Autodesk Inventor part; units mm, degrees
(part 2 of 2)
sketch "草圖6" plane through (-20.1844, 0, 27.5664) normal (0, 0, 1) x (1, 0, 0)
  line L0 (95.2719, 28.2499) -> (97.7719, 28.2499)
  line L1 (97.7719, 28.2499) -> (97.7719, 23.2499)
  line L2 (97.7719, 23.2499) -> (95.2719, 23.2499)
  line L3 (95.2719, 23.2499) -> (95.2719, 28.2499)
  line L4 (95.2719, 21.2499) -> (97.7719, 21.2499)
  line L5 (95.2719, 16.2499) -> (95.2719, 21.2499)
  line L6 (97.7719, 16.2499) -> (95.2719, 16.2499)
  line L7 (97.7719, 21.2499) -> (97.7719, 16.2499)
  line L8 (95.2719, 14.2499) -> (97.7719, 14.2499)
  line L9 (95.2719, 9.2499) -> (95.2719, 14.2499)
  line L10 (97.7719, 9.2499) -> (95.2719, 9.2499)
  line L11 (97.7719, 14.2499) -> (97.7719, 9.2499)
  line L12 (95.2719, 7.2499) -> (97.7719, 7.2499)
  line L13 (95.2719, 2.2499) -> (95.2719, 7.2499)
  line L14 (97.7719, 2.2499) -> (95.2719, 2.2499)
  line L15 (97.7719, 7.2499) -> (97.7719, 2.2499)
  line L16 (92.2719, 28.2499) -> (89.7719, 28.2499)
  line L17 (89.7719, 28.2499) -> (89.7719, 23.3875)
  line L18 (89.7719, 23.3875) -> (92.2719, 23.3875)
  line L19 (92.2719, 23.3875) -> (92.2719, 28.2499)
  line L20 (88.2719, 28.2499) -> (85.7719, 28.2499)
  line L21 (85.7719, 28.2499) -> (85.7719, 23.3875)
  line L22 (85.7719, 23.3875) -> (88.2719, 23.3875)
  line L23 (88.2719, 23.3875) -> (88.2719, 28.2499)
  line L24 (92.2719, 21.2499) -> (89.7719, 21.2499)
  line L25 (89.7719, 21.2499) -> (89.7719, 16.3875)
  line L26 (89.7719, 16.3875) -> (92.2719, 16.3875)
  line L27 (92.2719, 16.3875) -> (92.2719, 21.2499)
  line L28 (88.2719, 21.2499) -> (85.7719, 21.2499)
  line L29 (85.7719, 21.2499) -> (85.7719, 16.3875)
  line L30 (85.7719, 16.3875) -> (88.2719, 16.3875)
  line L31 (88.2719, 16.3875) -> (88.2719, 21.2499)
  line L32 (92.2719, 14.2499) -> (89.7719, 14.2499)
  line L33 (89.7719, 14.2499) -> (89.7719, 9.3875)
  line L34 (89.7719, 9.3875) -> (92.2719, 9.3875)
  line L35 (92.2719, 9.3875) -> (92.2719, 14.2499)
  line L36 (88.2719, 14.2499) -> (85.7719, 14.2499)
  line L37 (85.7719, 14.2499) -> (85.7719, 9.3875)
  line L38 (85.7719, 9.3875) -> (88.2719, 9.3875)
  line L39 (88.2719, 9.3875) -> (88.2719, 14.2499)
  line L40 (92.2719, 7.2499) -> (89.7719, 7.2499)
  line L41 (89.7719, 7.2499) -> (89.7719, 2.3875)
  line L42 (89.7719, 2.3875) -> (92.2719, 2.3875)
  line L43 (92.2719, 2.3875) -> (92.2719, 7.2499)
  line L44 (88.2719, 7.2499) -> (85.7719, 7.2499)
  line L45 (85.7719, 7.2499) -> (85.7719, 2.3875)
  line L46 (85.7719, 2.3875) -> (88.2719, 2.3875)
  line L47 (88.2719, 2.3875) -> (88.2719, 7.2499)
  line L48 (78.2719, 21.2499) -> (75.7719, 21.2499)
  line L49 (75.7719, 16.3875) -> (78.2719, 16.3875)
  line L50 (75.7719, 21.2499) -> (75.7719, 16.3875)
  line L51 (78.2719, 16.3875) -> (78.2719, 21.2499)
  line L52 (79.7719, 21.2499) -> (79.7719, 16.3875)
  line L53 (79.7719, 16.3875) -> (82.2719, 16.3875)
  line L54 (82.2719, 16.3875) -> (82.2719, 21.2499)
  line L55 (82.2719, 21.2499) -> (79.7719, 21.2499)
  line L56 (78.2719, 14.2499) -> (75.7719, 14.2499)
  line L57 (79.7719, 9.3875) -> (82.2719, 9.3875)
  line L58 (75.7719, 9.3875) -> (78.2719, 9.3875)
  line L59 (75.7719, 14.2499) -> (75.7719, 9.3875)
  line L60 (79.7719, 14.2499) -> (79.7719, 9.3875)
  line L61 (82.2719, 9.3875) -> (82.2719, 14.2499)
  line L62 (78.2719, 9.3875) -> (78.2719, 14.2499)
  line L63 (82.2719, 14.2499) -> (79.7719, 14.2499)
  line L64 (82.2719, 7.2499) -> (79.7719, 7.2499)
  line L65 (78.2719, 7.2499) -> (75.7719, 7.2499)
  line L66 (79.7719, 7.2499) -> (79.7719, 2.3875)
  line L67 (82.2719, 2.3875) -> (82.2719, 7.2499)
  line L68 (78.2719, 2.3875) -> (78.2719, 7.2499)
  line L69 (75.7719, 7.2499) -> (75.7719, 2.3875)
  line L70 (75.7719, 2.3875) -> (78.2719, 2.3875)
  line L71 (79.7719, 2.3875) -> (82.2719, 2.3875)
  line L72 (79.7719, 23.3875) -> (82.2719, 23.3875)
  line L73 (82.2719, 28.2499) -> (79.7719, 28.2499)
  line L74 (82.2719, 23.3875) -> (82.2719, 28.2499)
  line L75 (79.7719, 28.2499) -> (79.7719, 23.3875)
  line L76 (75.7719, 23.3875) -> (78.2719, 23.3875)
  line L77 (78.2719, 23.3875) -> (78.2719, 28.2499)
  line L78 (75.7719, 28.2499) -> (75.7719, 23.3875)
  line L79 (78.2719, 28.2499) -> (75.7719, 28.2499)
  line L80 (68.2719, 21.2499) -> (65.7719, 21.2499)
  line L81 (65.7719, 16.3875) -> (68.2719, 16.3875)
  line L82 (65.7719, 21.2499) -> (65.7719, 16.3875)
  line L83 (68.2719, 16.3875) -> (68.2719, 21.2499)
  line L84 (69.7719, 21.2499) -> (69.7719, 16.3875)
  line L85 (69.7719, 16.3875) -> (72.2719, 16.3875)
  line L86 (72.2719, 16.3875) -> (72.2719, 21.2499)
  line L87 (72.2719, 21.2499) -> (69.7719, 21.2499)
  line L88 (68.2719, 14.2499) -> (65.7719, 14.2499)
  line L89 (69.7719, 9.3875) -> (72.2719, 9.3875)
  line L90 (65.7719, 9.3875) -> (68.2719, 9.3875)
  line L91 (65.7719, 14.2499) -> (65.7719, 9.3875)
  line L92 (69.7719, 14.2499) -> (69.7719, 9.3875)
  line L93 (72.2719, 9.3875) -> (72.2719, 14.2499)
  line L94 (68.2719, 9.3875) -> (68.2719, 14.2499)
  line L95 (72.2719, 14.2499) -> (69.7719, 14.2499)
  line L96 (72.2719, 7.2499) -> (69.7719, 7.2499)
  line L97 (68.2719, 7.2499) -> (65.7719, 7.2499)
  line L98 (69.7719, 7.2499) -> (69.7719, 2.3875)
  line L99 (72.2719, 2.3875) -> (72.2719, 7.2499)
  line L100 (68.2719, 2.3875) -> (68.2719, 7.2499)
  line L101 (65.7719, 7.2499) -> (65.7719, 2.3875)
  line L102 (65.7719, 2.3875) -> (68.2719, 2.3875)
  line L103 (69.7719, 2.3875) -> (72.2719, 2.3875)
  line L104 (69.7719, 23.3875) -> (72.2719, 23.3875)
  line L105 (72.2719, 28.2499) -> (69.7719, 28.2499)
  line L106 (72.2719, 23.3875) -> (72.2719, 28.2499)
  line L107 (69.7719, 28.2499) -> (69.7719, 23.3875)
  line L108 (65.7719, 23.3875) -> (68.2719, 23.3875)
  line L109 (68.2719, 23.3875) -> (68.2719, 28.2499)
  line L110 (65.7719, 28.2499) -> (65.7719, 23.3875)
  line L111 (68.2719, 28.2499) -> (65.7719, 28.2499)
  line L112 (60.2719, 28.2499) -> (62.7719, 28.2499)
  line L113 (62.7719, 28.2499) -> (62.7719, 23.2499)
  line L114 (62.7719, 23.2499) -> (60.2719, 23.2499)
  line L115 (60.2719, 23.2499) -> (60.2719, 28.2499)
  line L116 (100, 30) -> (0, 30) projected
  line L117 (50, 30) -> (50, 0)
  line L118 (100, 0) -> (0, 0) projected
  line L119 (52.9784, 0) -> (46.9661, 0)
  line L120 (46.9661, 0) -> (46.9661, 21.3875)
  line L121 (46.9661, 21.3875) -> (52.9784, 21.3875)
  line L122 (52.9784, 21.3875) -> (52.9784, 0)
  line L123 (60.2719, 21.2499) -> (62.7719, 21.2499)
  line L124 (60.2719, 16.2499) -> (60.2719, 21.2499)
  line L125 (62.7719, 16.2499) -> (60.2719, 16.2499)
  line L126 (62.7719, 21.2499) -> (62.7719, 16.2499)
  line L127 (60.2719, 14.2499) -> (62.7719, 14.2499)
  line L128 (60.2719, 9.2499) -> (60.2719, 14.2499)
  line L129 (62.7719, 9.2499) -> (60.2719, 9.2499)
  line L130 (62.7719, 14.2499) -> (62.7719, 9.2499)
  line L131 (60.2719, 7.2499) -> (62.7719, 7.2499)
  line L132 (60.2719, 2.2499) -> (60.2719, 7.2499)
  line L133 (62.7719, 2.2499) -> (60.2719, 2.2499)
  line L134 (62.7719, 7.2499) -> (62.7719, 2.2499)
  line L135 (4.7281, 28.2499) -> (2.2281, 28.2499)
  line L136 (2.2281, 28.2499) -> (2.2281, 23.2499)
  line L137 (2.2281, 23.2499) -> (4.7281, 23.2499)
  line L138 (4.7281, 23.2499) -> (4.7281, 28.2499)
  line L139 (4.7281, 21.2499) -> (2.2281, 21.2499)
  line L140 (4.7281, 16.2499) -> (4.7281, 21.2499)
  line L141 (2.2281, 16.2499) -> (4.7281, 16.2499)
  line L142 (2.2281, 21.2499) -> (2.2281, 16.2499)
  line L143 (4.7281, 14.2499) -> (2.2281, 14.2499)
  line L144 (4.7281, 9.2499) -> (4.7281, 14.2499)
  line L145 (2.2281, 9.2499) -> (4.7281, 9.2499)
  line L146 (2.2281, 14.2499) -> (2.2281, 9.2499)
  line L147 (4.7281, 7.2499) -> (2.2281, 7.2499)
  line L148 (4.7281, 2.2499) -> (4.7281, 7.2499)
  line L149 (2.2281, 2.2499) -> (4.7281, 2.2499)
  line L150 (2.2281, 7.2499) -> (2.2281, 2.2499)
  line L151 (7.7281, 28.2499) -> (10.2281, 28.2499)
  line L152 (10.2281, 28.2499) -> (10.2281, 23.3875)
  line L153 (10.2281, 23.3875) -> (7.7281, 23.3875)
  line L154 (7.7281, 23.3875) -> (7.7281, 28.2499)
  line L155 (11.7281, 28.2499) -> (14.2281, 28.2499)
  line L156 (14.2281, 28.2499) -> (14.2281, 23.3875)
  line L157 (14.2281, 23.3875) -> (11.7281, 23.3875)
  line L158 (11.7281, 23.3875) -> (11.7281, 28.2499)
  line L159 (7.7281, 21.2499) -> (10.2281, 21.2499)
  line L160 (10.2281, 21.2499) -> (10.2281, 16.3875)
  line L161 (10.2281, 16.3875) -> (7.7281, 16.3875)
  line L162 (7.7281, 16.3875) -> (7.7281, 21.2499)
  line L163 (11.7281, 21.2499) -> (14.2281, 21.2499)
  line L164 (14.2281, 21.2499) -> (14.2281, 16.3875)
  line L165 (14.2281, 16.3875) -> (11.7281, 16.3875)
  line L166 (11.7281, 16.3875) -> (11.7281, 21.2499)
  line L167 (7.7281, 14.2499) -> (10.2281, 14.2499)
  line L168 (10.2281, 14.2499) -> (10.2281, 9.3875)
  line L169 (10.2281, 9.3875) -> (7.7281, 9.3875)
  line L170 (7.7281, 9.3875) -> (7.7281, 14.2499)
  line L171 (11.7281, 14.2499) -> (14.2281, 14.2499)
  line L172 (14.2281, 14.2499) -> (14.2281, 9.3875)
  line L173 (14.2281, 9.3875) -> (11.7281, 9.3875)
  line L174 (11.7281, 9.3875) -> (11.7281, 14.2499)
  line L175 (7.7281, 7.2499) -> (10.2281, 7.2499)
  line L176 (10.2281, 7.2499) -> (10.2281, 2.3875)
  line L177 (10.2281, 2.3875) -> (7.7281, 2.3875)
  line L178 (7.7281, 2.3875) -> (7.7281, 7.2499)
  line L179 (11.7281, 7.2499) -> (14.2281, 7.2499)
  line L180 (14.2281, 7.2499) -> (14.2281, 2.3875)
  line L181 (14.2281, 2.3875) -> (11.7281, 2.3875)
  line L182 (11.7281, 2.3875) -> (11.7281, 7.2499)
  line L183 (21.7281, 21.2499) -> (24.2281, 21.2499)
  line L184 (24.2281, 16.3875) -> (21.7281, 16.3875)
  line L185 (24.2281, 21.2499) -> (24.2281, 16.3875)
  line L186 (21.7281, 16.3875) -> (21.7281, 21.2499)
  line L187 (20.2281, 21.2499) -> (20.2281, 16.3875)
  line L188 (20.2281, 16.3875) -> (17.7281, 16.3875)
  line L189 (17.7281, 16.3875) -> (17.7281, 21.2499)
  line L190 (17.7281, 21.2499) -> (20.2281, 21.2499)
  line L191 (21.7281, 14.2499) -> (24.2281, 14.2499)
  line L192 (20.2281, 9.3875) -> (17.7281, 9.3875)
  line L193 (24.2281, 9.3875) -> (21.7281, 9.3875)
  line L194 (24.2281, 14.2499) -> (24.2281, 9.3875)
  line L195 (20.2281, 14.2499) -> (20.2281, 9.3875)
  line L196 (17.7281, 9.3875) -> (17.7281, 14.2499)
  line L197 (21.7281, 9.3875) -> (21.7281, 14.2499)
  line L198 (17.7281, 14.2499) -> (20.2281, 14.2499)
  line L199 (17.7281, 7.2499) -> (20.2281, 7.2499)
  line L200 (21.7281, 7.2499) -> (24.2281, 7.2499)
  line L201 (20.2281, 7.2499) -> (20.2281, 2.3875)
  line L202 (17.7281, 2.3875) -> (17.7281, 7.2499)
  line L203 (21.7281, 2.3875) -> (21.7281, 7.2499)
  line L204 (24.2281, 7.2499) -> (24.2281, 2.3875)
  line L205 (24.2281, 2.3875) -> (21.7281, 2.3875)
  line L206 (20.2281, 2.3875) -> (17.7281, 2.3875)
  line L207 (20.2281, 23.3875) -> (17.7281, 23.3875)
  line L208 (17.7281, 28.2499) -> (20.2281, 28.2499)
  line L209 (17.7281, 23.3875) -> (17.7281, 28.2499)
  line L210 (20.2281, 28.2499) -> (20.2281, 23.3875)
  line L211 (24.2281, 23.3875) -> (21.7281, 23.3875)
  line L212 (21.7281, 23.3875) -> (21.7281, 28.2499)
  line L213 (24.2281, 28.2499) -> (24.2281, 23.3875)
  line L214 (21.7281, 28.2499) -> (24.2281, 28.2499)
  line L215 (31.7281, 21.2499) -> (34.2281, 21.2499)
  line L216 (34.2281, 16.3875) -> (31.7281, 16.3875)
  line L217 (34.2281, 21.2499) -> (34.2281, 16.3875)
  line L218 (31.7281, 16.3875) -> (31.7281, 21.2499)
  line L219 (30.2281, 21.2499) -> (30.2281, 16.3875)
  line L220 (30.2281, 16.3875) -> (27.7281, 16.3875)
  line L221 (27.7281, 16.3875) -> (27.7281, 21.2499)
  line L222 (27.7281, 21.2499) -> (30.2281, 21.2499)
  line L223 (31.7281, 14.2499) -> (34.2281, 14.2499)
  line L224 (30.2281, 9.3875) -> (27.7281, 9.3875)
  line L225 (34.2281, 9.3875) -> (31.7281, 9.3875)
  line L226 (34.2281, 14.2499) -> (34.2281, 9.3875)
  line L227 (30.2281, 14.2499) -> (30.2281, 9.3875)
  line L228 (27.7281, 9.3875) -> (27.7281, 14.2499)
  line L229 (31.7281, 9.3875) -> (31.7281, 14.2499)
  line L230 (27.7281, 14.2499) -> (30.2281, 14.2499)
  line L231 (27.7281, 7.2499) -> (30.2281, 7.2499)
  line L232 (31.7281, 7.2499) -> (34.2281, 7.2499)
  line L233 (30.2281, 7.2499) -> (30.2281, 2.3875)
  line L234 (27.7281, 2.3875) -> (27.7281, 7.2499)
  line L235 (31.7281, 2.3875) -> (31.7281, 7.2499)
  line L236 (34.2281, 7.2499) -> (34.2281, 2.3875)
  line L237 (34.2281, 2.3875) -> (31.7281, 2.3875)
  line L238 (30.2281, 2.3875) -> (27.7281, 2.3875)
  line L239 (30.2281, 23.3875) -> (27.7281, 23.3875)
  line L240 (27.7281, 28.2499) -> (30.2281, 28.2499)
  line L241 (27.7281, 23.3875) -> (27.7281, 28.2499)
  line L242 (30.2281, 28.2499) -> (30.2281, 23.3875)
  line L243 (34.2281, 23.3875) -> (31.7281, 23.3875)
  line L244 (31.7281, 23.3875) -> (31.7281, 28.2499)
  line L245 (34.2281, 28.2499) -> (34.2281, 23.3875)
  line L246 (31.7281, 28.2499) -> (34.2281, 28.2499)
  line L247 (39.7281, 28.2499) -> (37.2281, 28.2499)
  line L248 (37.2281, 28.2499) -> (37.2281, 23.2499)
  line L249 (37.2281, 23.2499) -> (39.7281, 23.2499)
  line L250 (39.7281, 23.2499) -> (39.7281, 28.2499)
  line L251 (39.7281, 21.2499) -> (37.2281, 21.2499)
  line L252 (39.7281, 16.2499) -> (39.7281, 21.2499)
  line L253 (37.2281, 16.2499) -> (39.7281, 16.2499)
  line L254 (37.2281, 21.2499) -> (37.2281, 16.2499)
  line L255 (39.7281, 14.2499) -> (37.2281, 14.2499)
  line L256 (39.7281, 9.2499) -> (39.7281, 14.2499)
  line L257 (37.2281, 9.2499) -> (39.7281, 9.2499)
  line L258 (37.2281, 14.2499) -> (37.2281, 9.2499)
  line L259 (39.7281, 7.2499) -> (37.2281, 7.2499)
  line L260 (39.7281, 2.2499) -> (39.7281, 7.2499)
  line L261 (37.2281, 2.2499) -> (39.7281, 2.2499)
  line L262 (37.2281, 7.2499) -> (37.2281, 2.2499)
  line L263 (31.7281, 28.2499) -> (34.2281, 28.2499)
  line L264 (34.2281, 28.2499) -> (41.5067, 28.2499)
  point P0 (20.1844, 0)
  dimension "d230" = 2.5
  dimension "d231" = 5
  dimension "d234" = 7
  dimension "d239" = 2.5
  dimension "d242" = 4
  dimension "d245" = 7
  dimension "d250" = 10
  dimension "d256" = 3
  dimension "d258" = 2.5
  dimension "d259" = 5
  dimension "d260" = 3
  dimension "d263" = 7
  constraints: 526 end point, 128 symmetric about line, 9 equal length, 7 collinear, 7 horizontal, 4 perpendicular, 3 vertical, 2 midpoint, 1 point on line, 227 other
  measures "d230" distance of L1.end L2.end
  measures "d231" distance of L0.end L1.end
  measures "d234" distance of L0.end L4.end
  measures "d239" distance of L18.end L17.end
  measures "d242" distance of L16.start L20.start
  measures "d245" distance of L16.start L24.start
  measures "d250" distance of L28.start L48.start
  measures "d256" distance between parallel lines of L5 L27
  measures "d258" distance of L113.end L114.end
  measures "d259" distance of L114.end L112.start
  measures "d260" distance between parallel lines of L110 L113
  measures "d263" distance of L112.start L123.start
sketch "草圖7" plane through (0, 30, 0) normal (0, 1, 0) x (1, 0, 0)
  circle A0 centre (36.2637, -27.1141) radius 1.5
  line L0 (-20.1844, -27.5664) -> (79.8156, -27.5664) projected
  circle A1 centre (23.3676, -27.1141) radius 1.5
  point P0 (0, 0)
  dimension "d268" = 3
  constraints: 2 centre point
  measures "d268" diameter of A0
extrude "擠出6" add sketch "草圖7" along normal blind 1 and the other way blind 30
extrude "擠出7" cut sketch "草圖6" against normal blind 0.6 contours L0 L1 L2 L3 | L4 L7 L6 L5 | L8 L11 L10 L9 | L12 L15 L14 L13 | L19 L18 L17 L16 | L23 L22 L21 L20 | L27 L26 L25 L24 | L31 L30 L29 L28 | L35 L34 L33 L32 | L39 L38 L37 L36 | L43 L42 L41 L40 | L47 L46 L45 L44 | L51 L49 L50 L48 | L55 L54 L53 L52 | L62 L58 L59 L56 | L60 L63 L61 L57 | L67 L71 L66 L64 | L68 L70 L69 L65 | L75 L73 L74 L72 | L78 L79 L77 L76 | L83 L81 L82 L80 | L87 L86 L85 L84 | L94 L90 L91 L88 | L92 L95 L93 L89 | L99 L103 L98 L96 | L100 L102 L101 L97 | L107 L105 L106 L104 | L110 L111 L109 L108 | L112 L113 L114 L115 | L123 L126 L125 L124 | L127 L130 L129 L128 | L131 L134 L133 L132 | L138 L137 L136 L135 | L140 L141 L142 L139 | L144 L145 L146 L143 | L148 L149 L150 L147 | L151 L152 L153 L154 | L155 L156 L157 L158 | L159 L160 L161 L162 | L163 L164 L165 L166 | L167 L168 L169 L170 | L171 L172 L173 L174 | L175 L176 L177 L178 | L179 L180 L181 L182 | L183 L185 L184 L186 | L187 L188 L189 L190 | L191 L194 L193 L197 | L192 L196 L198 L195 | L199 L201 L206 L202 | L200 L204 L205 L203 | L207 L209 L208 L210 | L211 L212 L214 L213 | L215 L217 L216 L218 | L219 L220 L221 L222 | L223 L226 L225 L229 | L224 L228 L230 L227 | L231 L233 L238 L234 | L232 L236 L237 L235 | L239 L241 L240 L242 | L247 L250 L249 L248 | L243 L244 L246 L245 | L252 L253 L254 L251 | L256 L257 L258 L255 | L260 L261 L262 L259
ref_plane "工作平面1" through (79.8156, 0, -79.3336) normal (0, 0, -1) x (-1, 0, 0)
mirror "鏡射2" about plane through (79.8156, 0, -79.3336) normal (0, 0, -1) of "擠出7"
mirror "鏡射3" about plane through (79.8156, 0, -79.3336) normal (0, 0, -1) of "擠出6"
ref_plane "工作平面3" through (29.8156, 0, 27.5664) normal (1, 0, 0) x (0, 0, -1)
mirror "鏡射4" about plane through (29.8156, 0, 27.5664) normal (1, 0, 0) of "擠出4"
mirror "鏡射5" about plane through (29.8156, 0, 27.5664) normal (1, 0, 0) of "擠出5"
sketch "草圖8" plane through (0, 0, 0) normal (0, -1, 0) x (1, 0, 0)
  line L0 (79.8156, 27.5664) -> (79.8156, -34.4033) projected
  line L1 (-20.1844, -186.2336) -> (79.8156, -186.2336)
  line L2 (79.8156, -186.2336) -> (79.8156, 27.5664)
  line L3 (79.8156, 27.5664) -> (-20.1844, 27.5664)
  line L4 (-20.1844, 27.5664) -> (-20.1844, -186.2336)
  point P0 (0, 0)
  constraints: 8 end point, 2 parallel, 1 horizontal, 1 perpendicular
extrude "擠出8" add sketch "草圖8" along normal blind 8
sketch "草圖9" plane through (0, 30, 0) normal (0, 1, 0) x (1, 0, 0)
  line L0 (-20.1844, 186.2336) -> (-20.1844, 125.5723) projected
  line L1 (29.8156, 186.2336) -> (29.8156, 79.3336)
  line L2 (29.8156, 79.3336) -> (-20.1844, 79.3336)
  line L3 (1.8156, 8.3336) -> (1.8156, 150.3336)
  line L4 (1.8156, 150.3336) -> (57.8156, 150.3336)
  line L5 (57.8156, 150.3336) -> (57.8156, 8.3336)
  line L6 (57.8156, 8.3336) -> (1.8156, 8.3336)
  line L7 (1.8156, 8.3336) -> (57.8156, 150.3336) construction
  line L8 (1.8156, 150.3336) -> (57.8156, 8.3336) construction
  line L9 (29.8156, 79.3336) -> (29.8156, 99.3336)
  line L10 (29.8156, 99.3336) -> (65.8156, 99.3336)
  line L11 (65.8156, 99.3336) -> (65.8156, 134.3336)
  line L12 (65.8156, 134.3336) -> (29.8156, 134.3336)
  line L13 (29.8156, 134.3336) -> (29.8156, 99.3336)
  line L14 (29.8156, 134.3336) -> (29.8156, 99.3336)
  line L15 (29.8156, 99.3336) -> (-6.1844, 99.3336)
  line L16 (-6.1844, 99.3336) -> (-6.1844, 134.3336)
  line L17 (-6.1844, 134.3336) -> (29.8156, 134.3336)
  line L18 (29.8156, 79.3336) -> (29.8156, 59.3336)
  line L19 (29.8156, 59.3336) -> (29.8156, 24.3336)
  line L20 (29.8156, 24.3336) -> (65.8156, 24.3336)
  line L21 (65.8156, 24.3336) -> (65.8156, 59.3336)
  line L22 (65.8156, 59.3336) -> (29.8156, 59.3336)
  line L23 (29.8156, 59.3336) -> (29.8156, 24.3336)
  line L24 (29.8156, 24.3336) -> (-6.1844, 24.3336)
  line L25 (-6.1844, 24.3336) -> (-6.1844, 59.3336)
  line L26 (-6.1844, 59.3336) -> (29.8156, 59.3336)
  line L27 (0.8156, 59.3336) -> (58.8156, 59.3336)
  line L28 (58.8156, 59.3336) -> (58.8156, 99.3336)
  line L29 (58.8156, 99.3336) -> (0.8156, 99.3336)
  line L30 (0.8156, 99.3336) -> (0.8156, 59.3336)
  line L31 (0.8156, 59.3336) -> (58.8156, 99.3336) construction
  line L32 (58.8156, 59.3336) -> (0.8156, 99.3336) construction
  point P0 (0, 0)
  point P1 (1.8156, 134.3336)
  point P2 (1.8156, 24.3336)
  point P3 (57.8156, 24.3336)
  point P4 (57.8156, 134.3336)
  dimension "d279" = 106.9
  dimension "d280" = 142
  dimension "d281" = 56
  dimension "d282" = 20
  dimension "d283" = 36
  dimension "d284" = 35
  dimension "d285" = 36
  dimension "d286" = 20
  dimension "d287" = 35
  dimension "d288" = 36
  dimension "d289" = 36
  dimension "d290" = 58
  dimension "d291" = 40
  constraints: 64 end point, 12 parallel, 7 perpendicular, 4 midpoint, 2 collinear, 2 point on line, 1 horizontal, 1 vertical
  measures "d279" distance of L1.start L1.end
  measures "d280" distance of L3.start L3.end
  measures "d281" distance of L3.end L4.end
  measures "d282" distance of L1.end L9.end
  measures "d283" distance of L9.end L10.end
  measures "d284" distance of L11.end L10.end
  measures "d285" distance of L9.end L15.end
  measures "d286" distance of L1.end L18.end
  measures "d287" distance of L18.end L19.end
  measures "d288" distance of L20.end L19.end
  measures "d289" distance of L19.end L24.end
  measures "d290" distance of L27.start L27.end
  measures "d291" distance of L28.end L27.end
extrude "擠出9" add sketch "草圖9" along normal blind 0.01
sketch "草圖10" plane through (79.8156, 0, -34.4033) normal (1, 0, 0) x (0, 0, -1)
  line L0 (-61.9698, -8) -> (-61.9698, 30) projected
  line L1 (-61.9698, -8) -> (44.9302, -8)
  line L2 (-61.9698, -8) -> (151.8302, -8) projected
  line L3 (44.9302, -8) -> (44.9302, -0.5)
  line L4 (44.9302, -0.5) -> (49.9302, -0.5)
  line L5 (49.9302, -0.5) -> (49.9302, -8)
  line L6 (49.9302, -8) -> (44.9302, -8)
  line L7 (44.9302, -0.5) -> (44.9302, -8)
  line L8 (44.9302, -8) -> (39.9302, -8)
  line L9 (39.9302, -8) -> (39.9302, -0.5)
  line L10 (39.9302, -0.5) -> (44.9302, -0.5)
  point P0 (-34.4033, 0)
  dimension "d294" = 106.9
  dimension "d295" = 7.5
  dimension "d296" = 5
  dimension "d297" = 5
  constraints: 18 end point, 5 equal length, 3 perpendicular, 1 midpoint
  measures "d294" distance of L0.start L1.end
  measures "d295" distance of L1.end L3.end
  measures "d296" distance of L3.end L4.end
  measures "d297" distance of L1.end L8.end
extrude "擠出10" cut sketch "草圖10" against normal blind 2
mirror "鏡射6" about plane through (29.8156, 0, 27.5664) normal (1, 0, 0) of "擠出10"
ref_plane "工作平面2" through (79.8156, 0, -79.3336) normal (0, 0, -1) x (-1, 0, 0)
ref_plane "工作平面4" through (29.8156, 0, 27.5664) normal (1, 0, 0) x (0, 0, -1)
